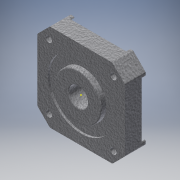
# Autodesk Inventor part: Part4
Saved by Autodesk Inventor 2019.3 (Build 233278000, 278)
## iProperties
Created: 2020-06-30
Part Number: Part4
Material: Allgemein
Document SubType Name: Modeling
Designer: IVAN
Density: 1 g/cm^3
Appearance: Aluminum Cast
Author: IVAN
Autodesk Inventor part; units mm, degrees
ref_plane "YZ Plane" through (0, 0, 0) normal (1, 0, 0) x (0, 1, 0)
ref_plane "XZ Plane" through (0, 0, 0) normal (0, 1, 0) x (-1, 0, 0)
ref_plane "XY Plane" through (0, 0, 0) normal (0, 0, 1) x (1, 0, 0)
sketch "Sketch1" plane through (0, 0, 0) normal (0, 1, 0) x (-1, 0, 0)
  line L0 (-21, -21) -> (21, -21)
  line L1 (21, -21) -> (21, 21)
  line L2 (21, 21) -> (-21, 21)
  line L3 (-21, 21) -> (-21, -21)
  line L4 (-21, -21) -> (21, 21) construction
  line L5 (21, -21) -> (-21, 21) construction
  point P0 (0, 0)
  dimension "d0" = 42
  dimension "d1" = 42
  constraints: 12 end point, 2 midpoint, 2 parallel, 1 horizontal, 1 perpendicular
  measures "d0" distance of L2.end L1.end
  measures "d1" distance of L1.end L0.end
extrude "Extrusion1" add sketch "Sketch1" along normal blind 8
sketch "Sketch2" plane through (0, 0, 0) normal (0, -1, 0) x (1, 0, 0)
  point P0 (0, 0)
chamfer "Chamfer1" distance 6 angle 45 4 edges at (-21, 4, 21) (21, 4, 21) (21, 4, -21) (-21, 4, -21)
sketch "Sketch3" plane through (0, 8, 0) normal (0, 1, 0) x (1, 0, 0)
  line L0 (-21, 15) -> (-15, 21) projected
  line L1 (-21, 15) -> (-21, -15) projected
  line L2 (-15, -21) -> (-21, -15) projected
  line L3 (-15, -21) -> (15, -21) projected
  line L4 (21, -15) -> (15, -21) projected
  line L5 (21, -15) -> (21, 15) projected
  line L6 (15, 21) -> (21, 15) projected
  line L7 (15, 21) -> (-15, 21) projected
  line L8 (-19.6609, -14.0495) -> (-13.6609, -20.0495)
  line L9 (-15, -21) -> (-21, -15) projected
  line L10 (-21, -15) -> (-19.8552, -13.8552)
  line L11 (-19.8552, -13.8552) -> (-19.6609, -14.0495)
  line L12 (-15, -21) -> (-13.8552, -19.8552)
  line L13 (-13.6609, -20.0495) -> (-13.1481, -20.5623)
  line L14 (-13.1481, -20.5623) -> (-13.5858, -21)
  line L15 (-19.8552, -13.8552) -> (-20.5623, -13.1481)
  line L16 (-20.5623, -13.1481) -> (-21, -13.5858)
  point P0 (0, 0)
  dimension "d11" = 1
  dimension "d12" = 1
  constraints: 16 end point, 4 perpendicular, 3 parallel, 3 point on line
  measures "d11" distance between parallel lines of L14 L12
  measures "d12" distance between parallel lines of L10 L16
extrude "Extrusion2" add sketch "Sketch3" along normal blind 2 contours L16 L15 L10 L1 | L10 L11 L8 L12 L2 | L12 L8 L13 L14 L3
mirror "Mirror1" about plane through (0, 0, 0) normal (0, 0, 1) of "Extrusion2"
mirror "Mirror2" about plane through (0, 0, 0) normal (1, 0, 0) of "Extrusion2", "Mirror1"
fillet "Fillet2" radius 1 8 edges at (15, 5, -21) (21, 5, -15) (21, 5, 15) (15, 5, 21) (-15, 5, 21) (-21, 5, 15) (-21, 5, -15) (-15, 5, -21)
fillet "Fillet3" radius 1 8 edges at (-21, 9, 13.5858) (-13.5858, 9, 21) (13.5858, 9, 21) (21, 9, 13.5858) (21, 9, -13.5858) (13.5858, 9, -21) (-13.5858, 9, -21) (-21, 9, -13.5858)
sketch "Sketch4" plane through (0, 0, 0) normal (0, -1, 0) x (1, 0, 0)
  circle A0 centre (0, 0) radius 16
  circle A1 centre (0, 0) radius 11
  dimension "d14" = 32
  dimension "d15" = 22
  constraints: 2 centre point, 2 coincident
  measures "d14" diameter of A0
  measures "d15" diameter of A1
extrude "Extrusion3" cut sketch "Sketch4" against normal blind 1
sketch "Sketch5" plane through (0, 0, 0) normal (0, -1, 0) x (1, 0, 0)
  circle A0 centre (0, 0) radius 11 projected
extrude "Extrusion4" add sketch "Sketch5" along normal blind 2
sketch "Sketch6" plane through (0, -2, 0) normal (0, -1, 0) x (1, 0, 0)
  circle A0 centre (0, 0) radius 4.5
  dimension "d20" = 9
  constraints: 1 centre point, 1 coincident
  measures "d20" diameter of A0
extrude "Extrusion5" cut sketch "Sketch6" against normal up to surface (10 mm away)
sketch "Sketch7" plane through (0, 0, 0) normal (0, -1, 0) x (1, 0, 0)
  point P0 (0, 0)
sketch "Sketch8" plane through (0, 0, 0) normal (0, -1, 0) x (1, 0, 0)
  circle A0 centre (-15.5, -15.5) radius 1.5
  line L0 (14.5858, -21) -> (-14.5858, -21) projected
  line L1 (-21, -14.5858) -> (-21, 14.5858) projected
  point P0 (0, 0)
  dimension "d23" = 3
  dimension "d24" = 5.5
  dimension "d25" = 5.5
  constraints: 1 centre point
  measures "d23" diameter of A0
  measures "d24" distance from line of L0 A0.centre
  measures "d25" distance from line of L1 A0.centre
extrude "Extrusion6" cut sketch "Sketch8" against normal blind 5
mirror "Mirror3" about plane through (0, 0, 0) normal (0, 0, 1) of "Extrusion6"
mirror "Mirror4" about plane through (0, 0, 0) normal (1, 0, 0) of "Extrusion6", "Mirror3"
fillet "Fillet4" radius 0.5 1 edges at (-11, -2, 0)
fillet "Fillet5" radius 0.5 1 edges at (-4.5, -2, 0)
equation "\"d12\" = d11"
equation "\"d25\" = d24"
body "Solid1"
